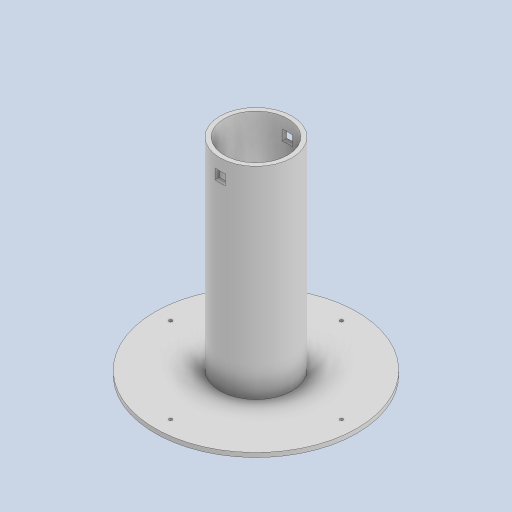
# Autodesk Inventor part: bottom card holder
Saved by Autodesk Inventor 2023 (Build 270158000, 158)
## iProperties
Created: 2023-06-01
Part Number: bottom card holder
Material: Generic
Document SubType Name: Modeling
Designer: cheng
Density: 1 g/cm^3
Appearance: Default
Author: cheng
Autodesk Inventor part; units mm, degrees
ref_plane "YZ Plane" through (0, 0, 0) normal (1, 0, 0) x (0, 1, 0)
ref_plane "XZ Plane" through (0, 0, 0) normal (0, 1, 0) x (-1, 0, 0)
ref_plane "XY Plane" through (0, 0, 0) normal (0, 0, 1) x (1, 0, 0)
sketch "Sketch1" plane through (0, 0, 0) normal (0, 1, 0) x (-1, 0, 0)
  circle A0 centre (0, 0) radius 70
  dimension "d0" = 140
  constraints: 1 centre point, 1 coincident
  measures "d0" diameter of A0
extrude "Extrusion1" add sketch "Sketch1" along normal blind 3
sketch "Sketch2" plane through (0, 3, 0) normal (0, 1, 0) x (1, 0, 0)
  circle A0 centre (0, 0) radius 25
  dimension "d3" = 50
  constraints: 1 centre point, 1 coincident
  measures "d3" diameter of A0
extrude "Extrusion2" add sketch "Sketch2" along normal blind 140
shell "Shell1" thickness 3 removed faces 1 at (4.976, 143, 4.8639)
sketch "Sketch3" plane through (0, 3, 0) normal (0, 1, 0) x (1, 0, 0)
  circle A0 centre (0, 0) radius 25 projected
  circle A1 centre (0, 0) radius 70 projected
  circle A2 centre (0, 0) radius 70 construction
  line L0 (-70, 0) -> (70, 0) construction
  line L1 (0, 70) -> (0, -70) construction
  line L2 (0, 0) -> (-49.4975, -49.4975) construction
  line L3 (0, 0) -> (49.4975, -49.4975) construction
  point P0 (0, -59.2377)
  point P1 (0, 59.2377)
  point P2 (-59.2377, 0)
  point P3 (59.2377, 0)
  dimension "d14" = 45
  dimension "d15" = 45
  constraints: 8 end point, 6 point on circle, 3 symmetric about line, 1 perpendicular, 1 point on line
  measures "d14" angle of L0 L2
  measures "d15" angle of L1 L3
hole "Hole1" at (0, 3, 59.2377) at (0, 3, -59.2377) at (59.2377, 3, 0) at (-59.2377, 3, 0) direction (0, -1, 0) diameter 2.3 end through all
sketch "Sketch4" plane through (0, 0, 0) normal (0, 0, 1) x (1, 0, 0)
  line L0 (25, 143) -> (-25, 143) projected
  line L1 (-25, 3) -> (25, 3) projected
  line L2 (70, 3) -> (-70, 3) projected
  line L3 (70, 0) -> (-70, 0) projected
  line L4 (25, 143) -> (-25, 143) construction
  line L5 (0, 143) -> (0, 0) construction
  line L6 (0, 143) -> (0, 0) construction
  line L7 (70, 3) -> (-70, 3) construction
  line L8 (-3.5, 135) -> (3.5, 135)
  line L9 (3.5, 135) -> (3.5, 128)
  line L10 (3.5, 128) -> (-3.5, 128)
  line L11 (-3.5, 128) -> (-3.5, 135)
  line L12 (-3.5, 135) -> (3.5, 128) construction
  line L13 (3.5, 135) -> (-3.5, 128) construction
  point P0 (0, 131.5)
  dimension "d18" = 7
  dimension "d19" = 7
  dimension "d23" = 125
  constraints: 16 end point, 3 midpoint, 2 parallel, 2 perpendicular, 1 horizontal, 1 point on line, 1 vertical
  measures "d18" distance of L8.end L9.end
  measures "d19" distance between parallel lines of L11 L9
  measures "d23" distance between parallel lines of L1 L10
extrude "Extrusion3" cut sketch "Sketch4" along normal mid plane 140
body "Solid1"
